Autodesk Fusion 360 part; units mm, degrees
(part 7 of 7)
equation "d2398 = CaseHeight - 16 mm"
named bodies: "Printed main housing", "Rear cavity cutting tool", "Upper sensor cavity cutting tool", "Single rear cover", "Retained factory frame", "Factory glass black border", "Active480x800 screen", "Guition PCB outline", "ESP32-P4 visual reference", "ESP32-C6 visual reference", "Memory visual reference", "Power inductor visual reference", "Power IC visual reference", "Factory USB visual reference", "FPC latch visual reference", "Expansion header visual reference", "GEN-M3-BHCS-L8-AF2 — joined head and shaft", "GEN-M3-HEATSET-OD4.2-L5 — hollow simplified insert", "PCB carrier plate", "Future shaped PCB", "Charger power zone", "Sensor analog zone", "Digital interface zone", "GEN-M2-SHCS-L7-AF1.5 — joined head and shaft", "GEN-M2-HEATSET-OD3.2-L4 — hollow simplified insert", "Removable display retainer plate", "GEN-M2-SHCS-L5-AF1.5 — joined head and shaft", "Measured occupied holder outer frame", "18650 reference cylinder - 18.2 diameter x 69 length", "Red battery disconnect reference body", "Red battery disconnect mating reference", "Button barrel", "External button bezel", "Button terminal block allowance", "Momentary push face", "Internal button nut reference", "Tiny flush metal bezel", "GCT8.44x2.66 throat R1.05", "GCT9.14x3.35 inner lip R1.39", "GCT9.64x3.86 gasket seat R1.65", "GCT external entry section", "GCT inner entry section", "USB printed frame floor", "Hidden USB common retaining bridge", "USB supported0.60mm daughterboard", "USB stainless main shell reference", "USB nose reference", "USB shell rear cavity simplified", "USB nose inner cavity simplified", "USB rear insulator", "USB LIM gasket reference", "USB gasket inner shell clearance", "USB visual contact stripe", "USB visual contact stripe (1)", "USB visual contact stripe (2)", "USB visual contact stripe (3)", "USB visual contact stripe (4)", "USB visual contact stripe (5)", "USB visual contact stripe (6)", "USB visual contact stripe (7)", "USB visual contact stripe (8)", "USB visual contact stripe (9)", "USB visual contact stripe (10)", "USB visual contact stripe (11)", "USB visual contact stripe (12)", "USB visual contact stripe (13)", "USB visual contact stripe (14)", "USB visual contact stripe (15)", "Bottom tiny bezel aperture with0.2mm clearance", "Manifold outer CO pocket", "Lid CO pocket", "Hand-tight adapter shoulder", "AO2 Ø29.3 dry body", "AO2 connector and wire origin allowance", "ZE07 PCB", "ZE07 CO can", "ZE07 header envelope", "MD62 full-size body", "MD62 full-length lead visual reference", "MD62 full-length lead visual reference (1)", "MD62 full-length lead visual reference (2)", "MD62 full-length lead visual reference (3)", "GYBMEP provisional PCB", "Humidity cap visual reference", "Breakout regulator height allowance", "Viewer-left inlet OD8 tube reference", "Viewer-right exhaust OD8 tube reference", "AO2 face seal allowance", "Potted harness closure reference"
